Autodesk Inventor part; units mm, degrees
(part 3 of 3)
extrude "Выдавливание1" add sketch "Эскиз1" along normal blind 2 contours A41 L1 L22 A0 | A0 L22 A844 A843 L1 A41 | L1 A844 L22 | A843 A844 L22 L154 L153 A385 A379 L156 A360 A386 A359 A388 A361 L157 L353 L354 L253 L379 L386 L385 L66 A129 A132 L65 A195 L5 L28 L170 A428 A425 L171 L12 L1 | L1 L12 L154 L22 A844 | L12 L171 L52 L339 L338 L337 L21 A847 L1 | L1 A848 L21 L337 L336 L335 L261 L310 L311 L145 A327 A351 A326 A348 A328 L143 A339 A347 L139 L140 L136 A331 A333 L135 A318 A332 A317 A329 A319 L134 L315 L316 L260 L321 L320 L319 L318 L317 L324 L323 L322 A88 L44 L313 A321 A330 A320 A336 A322 L137 A337 A335 L138 L142 L43 A80 L130 L129 A313 A307 L132 A288 A314 A287 A316 A289 L133 L265 L266 L47 L291 L298 L297 L296 L16 L115 L50 L49 L363 L362 L361 L368 L367 L366 L365 L263 L360 L357 L146 A357 A366 A356 A372 A358 L149 A373 A371 L150 L154 L12 | L154 L12 L152 L22 | L22 L152 A376 A378 L151 L155 A364 A384 A362 A387 A363 L157 L355 L356 L353 A361 A388 A359 A386 A360 L156 L153 A382 A380 L154 | A847 L21 A3 A38 L1 | L1 A38 A3 L21 A848 | L154 A374 A381 L150 L149 A358 A372 A356 A366 A357 L146 L357 L358 L359 A355 A365 A353 A368 A354 L147 L148 A377 A370 L152 L12 | A820 A819 | L52 A811 A103 A48 | A815 A816 | A163 A157 L77 A156 | A156 L77 A157 A163 | A158 A154 A156 L75 | L75 A156 A154 A158 | L183 L184 A153 A465 A151 A155 A152 L75 L34 | L183 L182 A464 A461 | L171 L170 L28 A20 A21 A53 L10 A62 L79 L78 A19 L80 L33 A60 A51 L32 A56 A61 A54 L31 A73 A70 A59 L38 | L152 L12 L216 A563 A560 A562 A571 A567 A565 A569 L217 A25 A22 L116 A47 L23 L428 L427 L426 L425 L22 | L22 L425 L424 L423 L247 L398 L399 L169 A399 A423 A398 A420 A400 L167 A411 A419 L163 L164 L160 A403 A405 L159 A390 A404 A389 A401 A391 L158 L403 L404 L245 L409 L408 L407 L64 A161 L76 A14 A17 L7 L189 A485 A474 L192 A483 A486 L8 A195 L65 L66 L385 L384 L383 L382 L381 L380 L379 L253 L354 L355 L157 A363 A387 A362 A384 A364 L155 A375 A383 L151 L152 | A380 A382 L153 L154 | A38 A3 L21 L1 | L1 L21 A3 A38 | L152 L148 A279 A369 L147 A354 A368 A353 A365 A355 L146 L359 L360 L263 L365 L364 L363 L49 A98 A95 L115 L12 | L154 L150 A381 A374 | A425 A428 L170 L171 | L171 L38 L39 L274 L273 L280 L279 L278 L277 L40 L272 L269 L122 A285 A294 A284 A300 A286 L125 A301 A299 L126 L130 A80 L43 L142 L141 A349 A343 L144 A324 A350 A323 A352 A325 L145 L309 L310 L261 L335 L342 L341 L340 L339 L52 | L425 L426 L427 L428 L23 L24 A40 A42 A707 L22 | L22 A44 L247 L423 L424 L425 | L152 L151 A378 A376 | L337 L338 L339 L52 A744 L21 | L21 A50 L261 L335 L336 L337 | L12 L217 A569 A565 A567 A571 A568 A562 A560 A563 L216 | A370 A377 L148 L152 | L339 L340 L341 L342 L335 L261 A39 L52 | L171 A430 A427 L172 A432 A429 L173 L35 L109 A258 A251 L113 A256 A259 L112 L62 L63 L119 A269 A272 L118 L59 A839 A840 L0 L48 A90 A93 L46 L128 L124 A295 A297 L123 A282 A296 A281 A293 A283 L122 L271 L272 L40 L277 L276 L275 L274 L39 A72 A75 L38 | L38 A59 A73 L37 A68 A55 L36 L35 L173 L172 L171 | L22 L247 A44 | L21 L261 A50 | A563 A560 A562 L216 | L216 A562 A560 A563 | A39 L261 L52 | A811 A812 | A75 A72 L39 L38 | L38 L37 A73 A59 | A59 A70 A73 L31 L38 | L171 L172 A427 A430 | A707 L24 L22 | L247 L24 A42 A40 | A40 A42 L429 L430 L423 L247 | L153 L156 A379 A385 | A744 L52 L21 | A371 A373 L149 L150 | L170 L173 L35 A69 A66 L36 A55 A71 A68 L29 A61 A58 A56 L32 A51 A60 L84 A180 A183 A179 A177 A181 L83 A175 A178 A174 A172 A176 L82 A20 L28 | L28 A10 A52 L5 A195 L88 L8 A13 A16 L7 A482 A480 A484 L191 A478 A481 A477 A475 A479 L190 A473 A476 L189 A17 A161 L64 L407 L406 L405 L412 L411 L410 L409 L245 L404 L401 L158 A393 A402 A392 A408 A394 L161 A409 A407 L162 L166 L165 A421 A415 L168 A396 A422 A395 A424 A397 L169 L397 L398 L247 L423 L430 L429 A42 A45 L23 L116 A278 A267 L117 L25 A32 A46 L18 A30 A33 L17 A34 A102 L19 L20 L121 A148 A273 A276 L120 A271 A274 L119 L70 A134 A139 L67 A136 A133 L68 L99 A229 A232 L112 A254 A257 L111 L71 L74 L73 L72 L109 L35 L173 A426 A431 L170 | L31 A73 L37 | L24 A40 A42 | A42 A40 L24 | A383 A375 L155 L151 | L12 L115 A268 A265 L116 A22 A25 | A569 A565 A567 L217 | L217 A567 A565 A569 | L148 L147 A369 A279 | L28 L5 A52 A10 | L28 L10 A53 A21 A20 | A20 L82 A170 A173 L81 A53 L27 L28 | A431 A426 L173 L170 | L31 A54 A57 L29 A68 L37 A73 | A40 L24 L23 L428 L429 A42 | L398 L397 L169 L399 | L23 A45 A42 L429 L428 | L310 L309 L145 L311 | L115 A95 L50 A831 A832 L16 L114 L61 L14 L15 A828 A827 L13 L12 | L12 L13 A22 L116 L115 | A571 A568 A562 | A562 L218 A567 A571 | L27 A53 L10 | L274 L275 L276 L277 L40 L39 | L39 A77 A74 L40 L277 L278 L279 L280 L273 L274 | L31 A61 L29 A57 A54 | A54 A61 L31 | L37 L36 A55 A68 | A68 L29 L37 | L172 L173 A429 A432 | L156 A359 A386 A360 | A360 A386 A359 L156 | L115 L50 A95 | A95 A98 L49 L50 L115 | L115 L116 A265 A268 | A568 A571 A567 L218 | L149 A356 A372 A358 | A358 A372 A356 L149 | L82 A176 A172 A174 A178 A175 L83 A181 A177 A179 A183 A180 L84 A60 L81 A53 A20 | A20 A53 L81 L82 | A53 L27 A60 L33 L80 L10 | A53 L81 A60 L27 | L39 L40 A74 A77 | A61 A54 L32 L31 | L31 L30 L29 A61 | A68 A71 A55 L36 L29 | L397 L400 L399 L169 | L169 A397 A424 A395 A422 A396 L168 L165 A418 A416 L166 A410 A417 L162 L161 A394 A408 A392 A402 A393 L158 L401 L402 L403 A391 A401 A389 A404 A390 L159 L160 A413 A406 L164 A412 A414 L163 L167 A400 A420 A398 A423 A399 L399 L400 L397 | A47 L116 L23 | L155 A362 A384 A364 | A364 A384 A362 L155 | L309 L312 L311 L145 | L145 A325 A352 A323 A350 A324 L144 L141 A346 A344 L142 L43 A672 A624 A683 A673 A684 A687 A689 A685 A690 A693 A82 L44 L314 L315 L134 A319 A329 A317 A332 A318 L135 L136 A341 A334 L140 A340 A342 L139 L143 A328 A348 A326 A351 A327 L311 L312 L309 | L13 A827 A828 L15 A26 A29 L14 A120 A27 L61 L114 L117 L25 A43 A47 L116 A22 | L115 A95 L50 | L147 A353 A368 A354 | A354 A368 A353 L147 | A195 L65 A225 A224 L5 | L5 A224 L88 A195 | L82 L81 A173 A170 | A176 A172 A174 L82 | L82 A174 A172 A176 | L80 L33 A65 L10 | A60 L81 A182 A171 L84 A51 L32 L27 | L27 L33 A60 | A61 A56 L32 A54 | L32 A56 A58 A61 L29 L30 | L169 A395 A424 A397 | A397 A424 A395 L169 | L169 A398 A423 A399 | A399 A423 A398 L169 | L116 A47 A43 L25 L23 | L23 L25 L117 L116 | L145 A323 A352 A325 | A325 A352 A323 L145 | L145 A326 A351 A327 | A327 A351 A326 L145 | A827 A828 L15 A24 A28 L13 | L13 A28 A24 L15 A828 A827 | A95 L115 L16 A832 A831 L50 | L65 A764 A696 | A224 A225 L8 A768 L6 L5 | L5 A718 A12 A9 A767 L8 A225 A224 | A195 L8 A225 L65 | A65 L33 L79 L10 | L10 L79 A62 | L80 L79 A19 L33 | L32 A51 A60 L33 | A60 L84 L81 | L35 L36 A66 A69 | L109 L71 L111 L112 A232 L98 A227 A230 L97 A248 A228 L108 L35 | L35 L108 A246 A249 L107 A244 A247 L106 L62 L112 L113 L109 | L116 L117 A267 A278 | A388 A361 L157 A359 | A359 L157 A361 A388 | A28 A24 L15 L13 | L13 L15 A24 A28 | L363 L364 L365 L263 L49 | L49 L263 L365 L366 L367 L368 L361 L362 L363 | A831 A832 L16 L50 | L50 L16 A832 A831 | L16 L296 L295 L294 L293 L292 L291 L47 L266 L267 L133 A291 A315 A290 A312 A292 L131 A303 A311 L127 L128 L46 L48 L0 A835 A836 L11 A119 A122 L60 L61 L114 A266 A263 L115 | A366 A357 L146 A356 | A356 L146 A357 A366 | L5 A12 A718 | A225 L8 A195 L88 | A132 A129 L66 L65 | L79 L33 L10 | L10 L34 L78 A19 A62 L79 | A19 L79 L33 | L81 L84 A171 A182 | L108 L97 L98 L99 L68 A6 A135 A771 L4 A67 A7 L35 | A780 A779 | A111 A108 A776 L55 | L35 L4 A772 A771 L68 L99 L100 A236 A233 L101 L102 L103 A241 A367 L104 L105 L106 L107 L108 | L109 L113 A251 A258 | A387 A363 L157 A362 | A362 L157 A363 A387 | L296 L297 L298 L291 L47 L16 | L16 A91 A100 L47 L291 L292 L293 L294 L295 L296 | A263 A266 L114 L115 | A365 A355 L146 A353 | A353 L146 A355 A365 | L5 L6 A767 A9 A718 A12 | A718 A9 A12 | L8 L7 A16 A13 | A178 A175 L83 A174 | A174 L83 A175 A178 | L33 L79 A19 L78 L34 | A62 A19 L78 L79 | A7 A67 L4 L35 | L108 L107 A249 A246 | A228 A248 L97 L108 | L272 L271 L122 L40 | L40 L122 L269 L272 | A422 A396 L168 A395 | A395 L168 A396 A422 | A420 A400 L167 A398 | A398 L167 A400 A420 | L117 A264 A277 L114 L61 A118 A121 L60 L11 A836 A835 L0 L48 L118 A275 A270 L121 A35 A37 L19 A31 A101 L17 L18 L25 | A350 A324 L144 A323 | A323 L144 A324 A350 | A348 A328 L143 A326 | A326 L143 A328 A348 | L15 L14 A29 A26 | L16 L47 A100 A91 | A9 A767 A718 | A767 A9 L6 A15 A11 L8 | L8 A11 A15 A697 A768 | L78 A19 L34 | L34 A19 L78 | L84 A179 A183 A180 | A180 A183 A179 L84 | A257 A254 L112 L111 | L25 L18 A46 A32 | L117 L114 A277 A264 | L353 L356 L355 L157 | L157 L355 L354 L353 | L357 L360 L359 L146 | L146 L359 L358 L357 | A768 A9 L6 | L6 A9 A767 | L8 L6 A15 A11 | A11 A15 L6 L8 | A697 A15 L6 A9 A768 | L385 L386 L379 L253 L66 | L66 L253 L379 L380 L381 L382 L383 L384 L385 | A764 A763 | L113 L112 A259 A256 | L271 L270 L40 L122 | L122 A283 A293 A281 A296 A282 L123 L124 A305 A298 L128 L46 L268 L265 L133 A289 A316 A287 A314 A288 L132 L129 A310 A308 L130 A78 A81 L236 L235 L41 A76 A79 L40 L270 L271 | L269 L270 L40 L41 A83 A80 L130 A302 A309 L126 L125 A286 A300 A284 A294 A285 L122 | L122 L40 L270 L269 | A482 L192 A483 L7 | A486 A483 L192 A482 | L7 L189 L190 A479 A475 A477 A481 A478 L191 A484 A480 A482 | A181 A177 A179 L83 | L83 A179 A177 A181 | A771 A135 L4 | L4 A5 A8 L68 A771 A772 | L107 L106 A247 A244 | A230 A227 L98 L97 | L122 A281 A293 A283 | A283 A293 A281 L122 | L122 A284 A294 A285 | A285 A294 A284 L122 | A415 A421 L165 L168 | L167 L163 A419 A411 | A343 A349 L141 L144 | L143 L139 A347 A339 | L14 L61 A27 A120 | L61 L60 A121 A118 | A483 L192 L189 L7 | A482 L191 A484 A480 | A480 A484 L191 A482 | A150 A463 L184 L183 | L4 L3 L68 A8 A5 | A771 L68 L3 L4 A135 | A135 A6 L68 A771 | L112 L98 A232 | A232 A229 L99 L112 | L18 L17 A33 A30 | L266 L265 L133 A89 L47 | L47 A89 A717 L46 L133 L267 L266 | L75 A151 A155 A152 | A152 A155 A151 L75 | L112 A242 A245 L105 A240 A243 A237 A239 L102 L55 L54 L53 L119 L63 A84 A126 L62 | L62 L106 A242 L112 | A79 A76 L41 L40 | A17 A14 A161 L9 L7 | L7 L9 A161 A17 | L189 L192 A474 A485 | A476 A473 L190 L189 | A126 A84 L63 L62 | L112 L105 A245 A242 | A242 L106 L112 | A296 A282 L123 A281 | A281 L123 A282 A296 | A300 A286 L125 A284 | A284 L125 A286 A300 | L165 L166 A416 A418 | A414 A412 L164 L163 | L141 L142 A344 A346 | A342 A340 L140 L139 | L47 A717 A89 | A89 A717 L47 | L265 L268 L46 A92 A89 L133 | L267 L268 L46 L128 A304 A306 L127 L131 A292 A312 A290 A315 A291 L133 | L133 A92 L46 L268 L267 | A122 A119 L11 L60 | A161 L9 A184 A185 L64 | L191 A477 A481 A478 | A478 A481 A477 L191 | L184 A151 A465 A153 | A153 A465 A151 L184 | A606 A608 A607 A610 | A610 A607 A608 A606 | A609 A602 A610 A604 | A604 A610 A602 A609 | A603 A600 A604 L228 | L228 A604 A600 A603 | L68 L67 L70 L119 A149 L53 A107 A104 L54 A109 A106 L55 L102 A235 A238 L112 A231 A234 L99 | A101 A31 L19 L51 L17 | A89 L133 L46 L47 A717 | L133 A287 A316 A289 | A289 A316 A287 L133 | A89 A92 L46 L133 | L133 L46 A92 | L133 A290 A315 A291 | A291 A315 A290 L133 | A161 A14 L9 | L64 A185 L76 A161 L212 L213 L214 | A133 A136 L67 L68 | A234 A231 L112 L99 | L235 A626 L236 A81 L41 | L17 L51 L19 A102 A34 | A14 A161 L76 A184 L9 | L407 L408 L409 L245 L64 | L64 L245 L409 L410 L411 L412 L405 L406 L407 | A756 A755 | A759 A760 | A185 A184 | L214 L213 L212 A161 | A479 A475 A477 L190 | L190 A477 A475 A479 | L112 A231 L100 | A783 A784 A753 L264 A125 L248 | A791 A792 | A799 A800 | L20 L256 A722 A720 | A796 A795 | A4 A137 L2 L69 | A138 A140 L69 L70 | A787 A788 | L53 L57 A105 A112 | L119 A149 L120 L121 A148 A35 L118 | L105 L112 A243 A240 | A81 A78 L130 L43 L42 L41 | L235 A626 | A297 A295 L124 L123 | L125 L126 A299 A301 | L166 L162 A417 A410 | A406 A413 L160 L164 | L231 A621 | L142 A338 A345 L138 L137 A322 A336 A320 A330 A321 L134 L313 L314 L44 A681 A678 A671 A676 A672 L43 | A334 A341 L136 L140 | A836 A835 L0 L11 | L11 A2 A123 L0 A835 A836 | A231 L112 A238 L101 L100 | L119 L118 A272 A269 | L104 A243 L112 | L41 L42 L43 L130 A80 A83 | A672 A676 A671 A678 A86 L43 | L43 A86 A82 A693 A688 A692 A690 A685 A689 A687 A682 A686 A684 A673 A683 A624 A670 A674 A672 | L43 A78 L130 A80 | A80 L130 A78 L43 | L142 L138 A345 A338 | A314 A288 L132 A287 | A287 L132 A288 A314 | A93 A90 L48 L46 | L128 L127 A306 A304 | A298 A305 L124 L128 | A312 A292 L131 A290 | A290 L131 A292 A312 | L11 L0 A123 A2 | L100 L101 A233 A236 | L112 L101 A238 | A238 A235 L102 L112 | L53 L54 A104 A107 | L104 L103 A237 L112 A243 | A86 A678 A679 A677 A681 L44 L43 | L43 L244 A86 | A676 A671 A678 A672 | A672 A678 A671 A676 | A674 A670 A624 A672 | L43 L130 A78 | A78 L130 L43 | A139 A134 L70 L67 | A784 L264 A753 | A753 L264 A784 | L248 A125 L264 A784 | A367 A241 L103 L104 | L112 L102 A239 A237 | A237 L103 L112 | A309 A302 L130 L126 | A407 A409 L161 L162 | L160 L159 A405 A403 | A37 A35 L121 L20 L19 | L43 L44 A681 A691 A680 A693 A82 A86 L244 | A308 A310 L129 L130 | L136 L135 A333 A331 | L0 A840 L59 L118 L48 | L404 L403 L158 L401 | L264 L248 A125 | L248 A125 | A678 A681 A677 A679 | A335 A337 L137 L138 | A307 A313 L129 L132 | A311 A303 L131 L127 | A840 A839 L59 A1 A116 L0 | L0 L59 A840 | L54 L55 A106 A109 | A274 A271 L120 L119 | L121 A35 L20 | L20 A35 L121 | L44 A82 A693 A680 A691 A681 | A683 A673 A684 A624 | A624 A684 A673 A683 | A116 A1 L59 L0 | L118 L121 A270 A275 | L403 L402 L401 L158 | L161 A392 A408 A394 | A394 A408 A392 L161 | L159 A389 A404 A390 | A390 A404 A389 L159 | A691 A680 A693 A681 | A681 A693 A680 A691 | L135 A317 A332 A318 | A318 A332 A317 L135 | L158 A389 A401 A391 | A391 A401 A389 L158 | L158 A392 A402 A393 | A393 A402 A392 L158 | A776 A108 L56 L55 | L55 L56 A108 A776 A775 | A693 A690 A692 A688 | L137 A320 A336 A322 | A322 A336 A320 L137 | A276 A273 L121 L120 | L256 A728 A804 L20 | L20 A804 A725 A721 A724 L254 A754 L256 | A722 L256 A720 | A720 L254 A731 A722 | L314 L313 L134 L44 | L44 L134 L315 L314 | A804 A728 A732 A730 A726 A729 L255 A723 A727 A725 | A754 L254 L256 | L256 A730 A804 A728 | A728 A732 A804 A730 L256 | L134 L313 L316 L44 | L44 L316 L315 L134 | A686 A682 A687 A684 | A329 A319 L134 A317 | A317 L134 A319 A329 | A804 A730 A732 A728 | A725 A727 A723 L255 A729 A726 A730 A732 A804 A803 | A690 A687 A689 A685 | A685 A689 A687 A690 | A330 A321 L134 A320 | A320 L134 A321 A330 | A804 A732 A730 | A725 L254 A724 A721 | A721 A724 L254 A725 | L44 L321 L260 L316 | A727 A723 L255 A725 | A725 L255 A723 A727 | L321 L322 A88 L44 | L44 A88 L260 L321 | A730 L255 A729 A726 | A726 A729 L255 A730 | A88 L322 L323 L324 L317 L318 L319 L320 L321 L260 L45 L44 | L44 L45 L260 A88 | A88 L322 | L89 A187 A201 L85 | L85 L86 A192 A188 A190 A197 A191 L87 A200 A196 A198 A202 A199 L89 | A189 A186 L86 L85 | L89 A198 A202 A199 | A199 A202 A198 L89 | A192 A188 A190 L86 | L86 A190 A188 A192 | A198 L87 A200 A196 | A196 A200 L87 A198 | A197 A191 L87 A190 | A190 L87 A191 A197 | A209 A280 A210 L90 | L90 A210 A280 A209 | L90 A206 A203 A204 A208 A205 L91 A211 A207 A209 A280 A210 | A206 A203 A204 L90 | L90 A204 A203 A206 | A209 L91 A211 A207 | A207 A211 L91 A209 | A208 A205 L91 A204 | A204 L91 A205 A208 | L92 L93 L94 | A260 A219 A261 L95 | L95 A261 A219 A260 | L95 A222 A218 A220 A226 A221 L96 A262 A223 A260 A219 A261 | A222 A218 A220 L95 | L95 A220 A218 A222 | A260 L96 A262 A223 | A223 A262 L96 A260 | A226 A221 L96 A220 | A220 L96 A221 A226 | A441 A437 A439 L176 | A448 A445 L178 A444 | A444 L178 A445 A448 | A446 A442 A444 L177 | L177 A444 A442 A446 | A443 A440 L177 A439 | A439 L177 A440 A443 | L176 A439 A437 A441 | A453 A449 A451 L179 | A460 A457 L181 A456 | A456 L181 A457 A460 | A458 A454 A456 L180 | L180 A456 A454 A458 | A455 A452 L180 A451 | A451 L180 A452 A455 | L179 A451 A449 A453 | L196 A472 | L195 A489 | L198 A495 | L198 L205 A530 A526 A528 A531 A529 L206 | A527 A524 L205 L198 | L206 A528 A531 A529 | A529 A531 A528 L206 | A530 A526 A528 L205 | L205 A528 A526 A530 | A582 A557 A583 L197 | L197 A583 A557 A582 | L197 L221 L222 A497 A580 A582 A558 A557 A583 | L221 A556 | A582 L222 A497 A580 | A580 A497 L222 A582 | A581 A578 L222 L221 | L202 A499 A510 L199 | L199 L200 A504 A500 A502 A506 A503 L201 A509 A505 A507 A511 A508 L202 | A501 A498 L200 L199 | L202 A507 A511 A508 | A508 A511 A507 L202 | A504 A500 A502 L200 | L200 A502 A500 A504 | A507 L201 A509 A505 | A505 A509 L201 A507 | A506 A503 L201 A502 | A502 L201 A503 A506 | A518 A513 A519 A512 | A512 A519 A513 A518 | A516 A514 A515 A512 | A512 A515 A514 A516 | A518 L203 A537 A521 | A575 A535 A577 A534 | A534 A577 A535 A575 | A573 A536 A550 A534 | A534 A550 A536 A573 | A585 A576 L220 A575 | A575 L220 A576 A585 | A545 L208 | L208 L209 A544 A540 A542 A546 A543 L210 | L210 A542 A546 A543 | A543 A546 A542 L210 | A541 A538 L209 L208 | A544 A540 A542 L209 | L209 A542 A540 A544 | A591 L224 A592 A572 | A592 L224 A591 A572 | A572 A591 L224 L226 L225 A590 A594 A592 A588 | L226 A589 | A594 A590 L225 A592 | A592 L225 A590 A594 | A593 A596 L225 L226 | A614 L229 A615 A611 | A617 A613 L230 A615 | A615 L230 A613 A617 | A615 L229 A614 A611 | A633 A638 A635 A637 | A633 A637 A635 A639 A634 A641 A642 A640 A644 A653 A643 A655 A650 A654 A652 A648 A651 A675 A645 A649 A647 A636 A646 A638 | A646 A636 A647 A638 | A638 A647 A636 A646 | A639 A634 A641 A635 | A635 A641 A634 A639 | A641 A644 A640 A642 | A649 A645 A675 A647 | A675 A652 A648 A651 | A651 A648 A652 A675 | A653 A643 A655 A644 | A644 A655 A643 A653 | A654 A650 A655 A652 | L238 A659 | L242 A663 | A808 A807 | A824 A823
sketch "Эскиз4" plane through (0, 0, 0) normal (0, 0, -1) x (-1, 0, 0)
  line L0 (13.871, 36.947) -> (13.871, -1.143) projected
  line L1 (13.871, -1.143) -> (-46.4987, -1.143) construction
  line L2 (-46.4987, -1.143) -> (-46.4987, 37.2069) construction
  line L3 (-46.4987, 37.2069) -> (13.871, 37.2069) construction
  line L4 (13.871, 37.2069) -> (13.871, -1.143) construction
  point P0 (0, 0)
  constraints: 2 other
